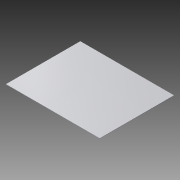
# Autodesk Inventor part: UltibotsHeatSpreader230x290
Saved by Autodesk Inventor 2016 (Build 200138000, 138)
## iProperties
Created: 2014-12-21
Part Number: UltibotsHeatSpreader230x290
Material: Aluminum 6061
Document SubType Name: Modeling
Designer: Jack
Density: 2.7 g/cm^3
Appearance: Aluminum - Flat
Mass: 288.144 g
Surface Area: 1350.64 cm^2
Volume: 106.72 cm^3
Catalog Web Link: http://www.ultibots.com/heat-spreader-230mm-x-290mm/
Vendor: Ultibots
Author: Jack
Autodesk Inventor part; units mm, degrees
ref_plane "YZ Plane" through (0, 0, 0) normal (1, 0, 0) x (0, 1, 0)
ref_plane "XZ Plane" through (0, 0, 0) normal (0, 1, 0) x (-1, 0, 0)
ref_plane "XY Plane" through (0, 0, 0) normal (0, 0, 1) x (1, 0, 0)
sketch "Sketch1" plane through (0, 0, 0) normal (0, 0, 1) x (1, 0, 0)
  line L0 (0, 0) -> (290, 0)
  line L1 (290, 0) -> (290, 230)
  line L2 (290, 230) -> (0, 230)
  line L3 (0, 230) -> (0, 0)
  dimension "d0" = 290
  dimension "d1" = 230
  constraints: 8 end point, 2 parallel, 1 horizontal, 1 perpendicular
  measures "d0" distance of L2.end L1.end
  measures "d1" distance of L1.end L0.end
extrude "Extrusion1" add sketch "Sketch1" along normal blind 1.6
body "Solid1"
